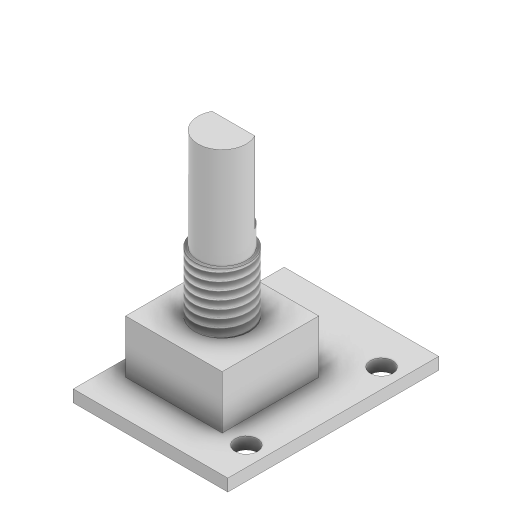
# Autodesk Inventor part: 編碼器
Saved by Autodesk Inventor 2024 (Build 280153000, 153)
## iProperties
Created: 2024-05-19
Part Number: 編碼器
Material: 一般
Document SubType Name: Modeling
Designer: rumse
Density: 1 g/cm^3
Appearance: 預設
Author: rumse
Autodesk Inventor part; units mm, degrees
ref_plane "YZ Plane" through (0, 0, 0) normal (1, 0, 0) x (0, 1, 0)
ref_plane "XZ Plane" through (0, 0, 0) normal (0, 1, 0) x (-1, 0, 0)
ref_plane "XY Plane" through (0, 0, 0) normal (0, 0, 1) x (1, 0, 0)
sketch "草圖2" plane through (0, 0, 0) normal (0, 1, 0) x (-1, 0, 0)
  line L0 (0, 0) -> (19.2, 0)
  line L1 (19.2, 0) -> (19.2, -26.2)
  line L2 (19.2, -26.2) -> (0, -26.2)
  line L3 (0, -26.2) -> (0, 0)
  dimension "d4" = 26.2
  dimension "d5" = 19.2
  constraints: 8 end point, 2 parallel, 1 horizontal, 1 perpendicular
  measures "d4" distance of L0.end L1.end
  measures "d5" distance of L1.end L2.end
extrude "擠出2" add sketch "草圖2" along normal blind 1.5
sketch "草圖3" plane through (0, 1.5, 0) normal (0, 1, 0) x (1, 0, 0)
  line L0 (-19.2, 0) -> (0, 0) projected
  line L1 (-19.2, 26.2) -> (-19.2, 0) projected
  line L2 (-17.2, 4.5) -> (-5.2, 4.5)
  line L3 (-5.2, 4.5) -> (-5.2, 16.5)
  line L4 (-5.2, 16.5) -> (-17.2, 16.5)
  line L5 (-17.2, 16.5) -> (-17.2, 4.5)
  dimension "d8" = 4.5
  dimension "d9" = 2
  dimension "d10" = 12
  dimension "d11" = 12
  constraints: 8 end point, 2 parallel, 1 horizontal, 1 perpendicular
  measures "d8" distance from line of L2.start L0
  measures "d9" distance from line of L2.start L1
  measures "d10" distance of L4.end L2.start
  measures "d11" distance of L2.start L2.end
extrude "擠出3" add sketch "草圖3" along normal blind 6.6
sketch "草圖4" plane through (0, 8.1, 0) normal (0, 1, 0) x (1, 0, 0)
  line L0 (-5.2, 4.5) -> (-5.2, 16.5) projected
  line L1 (-5.2, 16.5) -> (-17.2, 16.5) projected
  line L2 (-17.2, 16.5) -> (-17.2, 4.5) projected
  line L3 (-17.2, 4.5) -> (-5.2, 4.5) projected
  circle A0 centre (-11.2, 10.5) radius 3.4
  point P0 (0, 0)
  dimension "d14" = 6
  dimension "d15" = 6
  dimension "d16" = 6.8
  constraints: 1 centre point, 1 coincident
  measures "d14" distance from line of L2 point (-11.2, 10.5)
  measures "d15" distance from line of L3 point (-11.2, 10.5)
  measures "d16" diameter of A0
extrude "擠出4" add sketch "草圖4" along normal blind 7.46 contours A0
sketch "草圖5" plane through (-11.2, 15.56, -10.5) normal (0, 1, 0) x (1, 0, 0)
  circle A0 centre (0, 0) radius 3.4 projected
  circle A1 centre (0, 0) radius 3
  point P0 (11.2, -10.5)
  dimension "d19" = 6
  constraints: 1 centre point, 1 coincident
  measures "d19" diameter of A1
extrude "擠出5" add sketch "草圖5" along normal blind 12.54 contours A1
thread "螺紋1" size "M7x1" class "6g" standard "ANSI Metric M Profile" full length
sketch "草圖6" plane through (-11.2, 28.1, -10.5) normal (0, 1, 0) x (1, 0, 0)
  line L0 (-3, 1.4) -> (3, 1.4)
  line L1 (3, 1.4) -> (3, 3)
  line L2 (3, 3) -> (-3, 3)
  line L3 (-3, 3) -> (-3, 1.4)
  circle A0 centre (0, 0) radius 3 projected
  point P0 (11.2, -10.5)
  point P1 (0, 3)
  point P2 (0, 3)
  point P3 (-3, 0)
  dimension "d24" = 1.6
  dimension "d25" = 6
  constraints: 8 end point, 3 horizontal alignment, 3 point on circle, 2 parallel, 1 coincident, 1 horizontal, 1 perpendicular, 1 tangent, 1 vertical alignment
  measures "d24" distance of L0.end L1.end
  measures "d25" distance of L1.end L2.end
extrude "擠出6" cut sketch "草圖6" against normal blind 10 contours L3 L2 A0 L0 | A0 L0 | A0 L2 L1 L0 picked at (0.7632, 1.5795)
sketch "草圖7" plane through (0, 0, 0) normal (0, -1, 0) x (1, 0, 0)
  circle A0 centre (-2.4, -4.7) radius 1.4
  circle A1 centre (-2.4, -21.5) radius 1.4
  line L0 (0, 0) -> (0, -26.2) projected
  line L1 (-19.2, 0) -> (0, 0) projected
  dimension "d29" = 16.8
  dimension "d30" = 2.8
  dimension "d31" = 2.4
  dimension "d33" = 4.7
  constraints: 2 centre point, 1 equal radius, 1 vertical alignment
  measures "d29" distance of A1.centre A0.centre
  measures "d30" diameter of A0
  measures "d31" distance from line of L0 A0.centre
  measures "d33" distance from line of L1 A0.centre
extrude "擠出7" cut sketch "草圖7" against normal up to surface (1.5 mm away)
